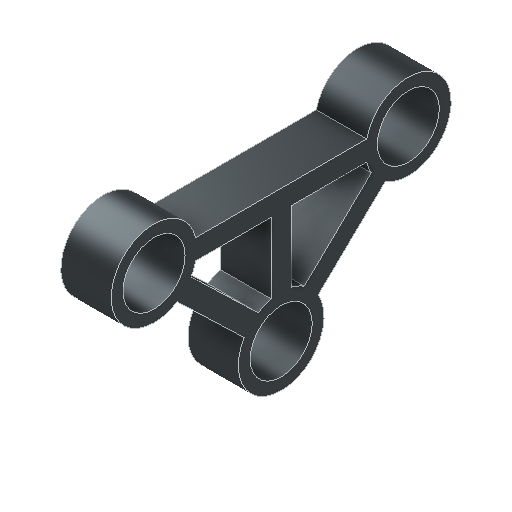
# Autodesk Inventor part: TriangleLink_CBF
Saved by Autodesk Inventor 2026.2 (Build 302298000, 298)
## iProperties
Created: 2025-12-27
Part Number: TriangleLink_CBF
Material: ABS 塑膠
Document SubType Name: Modeling
Designer: Hsiangyu
Density: 1.06 g/cm^3
Appearance: 鐵灰色
Author: Hsiangyu
Autodesk Inventor part; units mm, degrees
ref_plane "YZ Plane" through (0, 0, 0) normal (1, 0, 0) x (0, 1, 0)
ref_plane "XZ Plane" through (0, 0, 0) normal (0, 1, 0) x (-1, 0, 0)
ref_plane "XY Plane" through (0, 0, 0) normal (0, 0, 1) x (1, 0, 0)
sketch "草圖1" plane through (0, 0, 0) normal (1, 0, 0) x (0, 1, 0)
  line L0 (0, 0) -> (24.2691, 25.2193)
  line L1 (24.2691, 25.2193) -> (24.2691, -25.2193)
  line L2 (24.2691, -25.2193) -> (0, 0)
  line L3 (0, 0) -> (24.2691, 0)
  circle A0 centre (24.2691, 25.2193) radius 6.15
  circle A1 centre (24.2691, -25.2193) radius 6.15
  circle A2 centre (0, 0) radius 6.15
  circle A3 centre (24.2691, 25.2193) radius 8.5
  circle A4 centre (24.2691, -25.2193) radius 8.5
  circle A5 centre (0, 0) radius 8.5
  line L4 (26.2691, 16.9579) -> (26.2691, -16.9579)
  line L5 (22.2691, 16.9579) -> (22.2691, -16.9579)
  line L6 (17.0995, 20.6534) -> (4.2873, 7.3395)
  line L7 (4.2873, -7.3395) -> (17.0995, -20.6534)
  line L8 (19.9817, 17.8798) -> (7.1695, 4.5659)
  line L9 (7.1695, -4.5659) -> (19.9817, -17.8798)
  line L10 (8.2614, 2) -> (24.2691, 2)
  line L11 (8.2614, -2) -> (24.2691, -2)
  point P0 (22.2691, 2)
  point P1 (22.2691, -2)
  dimension "d0" = 92.2
  dimension "d1" = 35
  dimension "d2" = 35
  dimension "d3" = 12.3
  dimension "d4" = 17
  dimension "d5" = 2
  dimension "d6" = 2
  dimension "d7" = 2
  dimension "d8" = 2
  dimension "d9" = 2
  dimension "d10" = 2
  dimension "d13" = 2
  dimension "d14" = 2
  constraints: 24 end point, 14 point on circle, 6 centre point, 6 coincident, 4 equal radius, 2 perpendicular, 2 point on line, 2 vertical, 1 midpoint, 1 parallel
  measures "d0" angle of L2 L0
  measures "d1" distance of L0.start L0.end
  measures "d2" distance of L1.end L0.start
  measures "d3" diameter of A0
  measures "d4" diameter of A3
  measures "d5" distance between parallel lines of L4 L1
  measures "d6" distance between parallel lines of L5 L1
  measures "d7" distance between parallel lines of L0 L8
  measures "d8" distance between parallel lines of L6 L0
  measures "d9" distance between parallel lines of L9 L2
  measures "d10" distance between parallel lines of L2 L7
  measures "d13" distance from line of L0.start L10
  measures "d14" distance from line of L0.start L11
extrude "擠出1" add sketch "草圖1" along normal blind 10 contours A2 L2 A5 L0 | L0 A5 L3 A2 | A2 L3 A5 L2 | A5 L6 A3 L0 | L0 A3 L8 A5 | A5 L9 A4 L2 | L2 A4 L7 A5 | A5 L10 L5 L3 | L3 L5 L11 A5 | A3 L1 A0 L0 | L0 A0 L1 A3 | A4 L1 A1 L2 | L2 A1 L1 A4 | L5 L10 L1 L3 | L3 L1 L11 L5 | L1 A3 L4 A4 | L5 A3 L1 L10 | L11 L1 A4 L5
equation "\"d6\" = d5"
equation "\"d7\" = d5"
equation "\"d8\" = d5"
equation "\"d9\" = d5"
equation "\"d10\" = d5"
equation "\"d13\" = d5"
equation "\"d14\" = d5"
